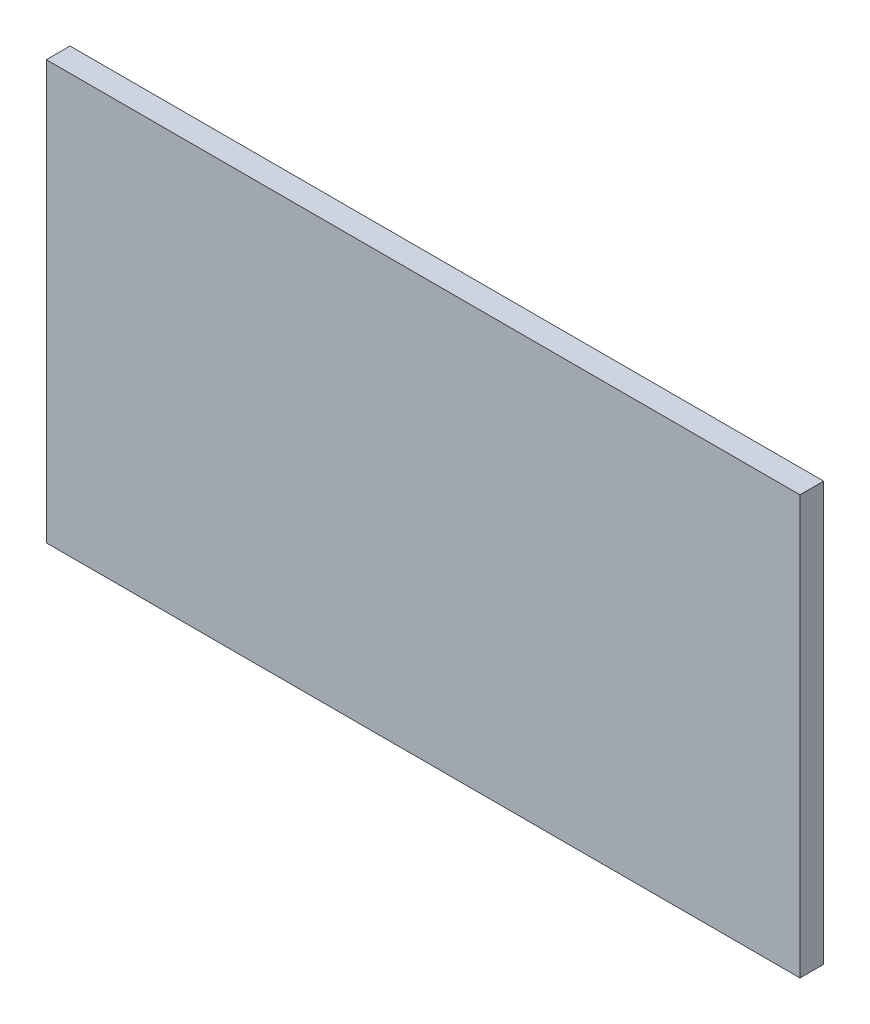
# Autodesk Inventor part: tapa acrilica
Saved by Autodesk Inventor 2017 (Build 210142000, 142)
## iProperties
Part Number: tapa acrilica
Material: Genérico
Document SubType Name: Modeling
Designer: Leo
Density: 1 g/cm^3
Appearance: Claro
Author: Leo
Autodesk Inventor part; units mm, degrees
ref_plane "YZ Plane" through (0, 0, 0) normal (1, 0, 0) x (0, 1, 0)
ref_plane "XZ Plane" through (0, 0, 0) normal (0, 1, 0) x (-1, 0, 0)
ref_plane "XY Plane" through (0, 0, 0) normal (0, 0, 1) x (1, 0, 0)
sketch "Boceto1" plane through (0, 0, 0) normal (0, 0, 1) x (1, 0, 0)
  line L0 (-76.2, -33) -> (-76.2, 33) construction
  arc A0 (-76.2, 33) -> (-84.2, 41) centre (-84.2, 33) ccw construction
  line L1 (-84.2, 41) -> (-229.1, 41) construction
  arc A1 (-229.1, 41) -> (-237.1, 33) centre (-229.1, 33) ccw construction
  line L2 (-237.1, 33) -> (-237.1, -33) construction
  arc A2 (-237.1, -33) -> (-229.1, -41) centre (-229.1, -33) ccw construction
  line L3 (-229.1, -41) -> (-84.2, -41) construction
  arc A3 (-84.2, -41) -> (-76.2, -33) centre (-84.2, -33) ccw construction
  line L4 (-61.2, -53) -> (-252.1, -53)
  line L5 (-252.1, -53) -> (-252.1, 53)
  line L6 (-252.1, 53) -> (-61.2, 53)
  line L7 (-61.2, 53) -> (-61.2, -53)
  point P0 (0, 0)
  point P1 (-156.65, -41)
  point P2 (-156.65, -53)
  point P3 (-76.2, 0)
  point P4 (-61.2, 0)
  dimension "d0" = 15
  dimension "d1" = 106
  constraints: 8 end point, 4 midpoint, 2 parallel, 1 horizontal, 1 horizontal alignment, 1 perpendicular, 1 vertical alignment
  measures "d0" distance between parallel lines of L7 L0
  measures "d1" distance between parallel lines of L6 L4
extrude "Extrusión1" add sketch "Boceto1" along normal blind 6
